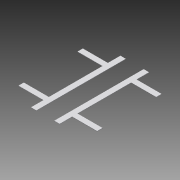
# Autodesk Inventor part: Aluminum Board
Saved by Autodesk Inventor 2014 SP1 (Build 180222100, 222)
## iProperties
Created: 2014-01-18
Part Number: Aluminum Board
Material: Generic
Document SubType Name: Modeling
Designer: Paul
Density: 1 g/cm^3
Appearance: Aluminum - Polished
Author: Paul
Autodesk Inventor part; units mm, degrees
ref_plane "YZ Plane" through (0, 0, 0) normal (1, 0, 0) x (0, 1, 0)
ref_plane "XZ Plane" through (0, 0, 0) normal (0, 1, 0) x (-1, 0, 0)
ref_plane "XY Plane" through (0, 0, 0) normal (0, 0, 1) x (1, 0, 0)
sketch "Sketch1" plane through (0, 0, 0) normal (0, 1, 0) x (-1, 0, 0)
  line L0 (0, 0) -> (0, 88.9)
  line L1 (0, 88.9) -> (-177.8, 88.9)
  line L2 (-177.8, 88.9) -> (-177.8, 546.1)
  line L3 (-177.8, 546.1) -> (0, 546.1)
  line L4 (0, 546.1) -> (0, 635)
  line L5 (0, 635) -> (203.2, 635)
  line L6 (203.2, 635) -> (203.2, 546.1)
  line L7 (203.2, 546.1) -> (381, 546.1)
  line L8 (381, 546.1) -> (381, 88.9)
  line L9 (381, 88.9) -> (203.2, 88.9)
  line L10 (203.2, 88.9) -> (203.2, 0)
  line L11 (203.2, 0) -> (0, 0)
  dimension "d0" = 88.9
  dimension "d1" = 177.8
  dimension "d2" = 88.9
  dimension "d3" = 177.8
  dimension "d4" = 177.8
  dimension "d5" = 88.9
  dimension "d6" = 177.8
  dimension "d7" = 88.9
  dimension "d8" = 558.8
  dimension "d9" = 635
  constraints: 24 end point, 8 parallel, 2 collinear, 1 perpendicular, 1 vertical
  measures "d0" distance of L9.end L10.end
  measures "d1" distance of L8.end L9.end
  measures "d2" distance of L5.end L6.end
  measures "d3" distance of L6.end L7.end
  measures "d4" distance of L2.end L3.end
  measures "d5" distance of L3.end L4.end
  measures "d6" distance of L0.end L1.end
  measures "d7" distance of L0.start L0.end
  measures "d8" distance between parallel lines of L8 L2
  measures "d9" distance between parallel lines of L11 L5
extrude "Extrusion1" add sketch "Sketch1" along normal blind 3.175
sketch "Sketch2" plane through (0, 0, 0) normal (0, -1, 0) x (1, 0, 0)
  line L0 (0, 0) -> (0, 88.9) projected
  line L1 (0, 546.1) -> (0, 635) projected
  line L2 (0, 635) -> (-203.2, 635) projected
  line L3 (-203.2, 546.1) -> (-381, 546.1) projected
  line L4 (-381, 88.9) -> (-203.2, 88.9) projected
  line L5 (-203.2, 0) -> (0, 0) projected
  line L6 (-38.1, 635) -> (-165.1, 635)
  line L7 (-165.1, 635) -> (-165.1, 0)
  line L8 (-165.1, 0) -> (-38.1, 0)
  line L9 (-38.1, 0) -> (-38.1, 635)
  line L10 (0, 546.1) -> (0, 88.9)
  line L11 (-203.2, 546.1) -> (-203.2, 88.9)
  line L12 (-203.2, 508) -> (-381, 508)
  line L13 (-381, 508) -> (-381, 127)
  line L14 (-381, 127) -> (-203.2, 127)
  line L15 (-203.2, 127) -> (-203.2, 508)
  line L16 (0, 508) -> (177.8, 508)
  line L17 (177.8, 508) -> (177.8, 127)
  line L18 (177.8, 127) -> (0, 127)
  line L19 (0, 127) -> (0, 508)
  dimension "d12" = 127
  dimension "d13" = 38.1
  dimension "d14" = 38.1
  dimension "d15" = 38.1
  dimension "d16" = 177.8
  dimension "d17" = 177.8
  constraints: 28 end point, 7 parallel, 4 point on line, 3 horizontal, 3 perpendicular, 1 collinear
  measures "d12" distance of L8.end L7.end
  measures "d13" distance between parallel lines of L1 L9
  measures "d14" distance between parallel lines of L3 L12
  measures "d15" distance between parallel lines of L4 L14
  measures "d16" distance between parallel lines of L13 L15
  measures "d17" distance of L17.end L18.end
extrude "Extrusion2" cut sketch "Sketch2" against normal blind 25.4 contours L5 L7 L2 L9 | L10 L16 L17 L18 | L11 L14 L13 L12
body "Solid1"
